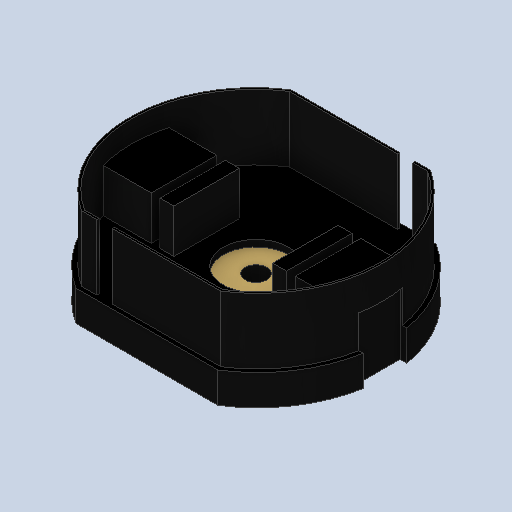
# Autodesk Inventor part: Base
Saved by Autodesk Inventor 2022.2 (Build 262287000, 287)
## iProperties
Created: 2021-01-16
Part Number: Base
Material: Ouro
Document SubType Name: Modeling
Designer: João
Density: 19.3 g/cm^3
Appearance: Suave - Preto
Mass: 3.82351 g
Surface Area: 5.41035 cm^2
Volume: 0.198109 cm^3
Author: João
Autodesk Inventor part; units mm, degrees
sketch "Esboço1" plane through (0, 0, 0) normal (0, 1, 0) x (-1, 0, 0)
  line L0 (3.25, 5) -> (-3.25, 5)
  line L1 (-3.25, -5) -> (3.25, -5)
  arc A0 (3.25, -5) -> (3.25, 5) centre (0.0795, 0) ccw
  arc A1 (-3.25, 5) -> (-3.25, -5) centre (-0.0795, 0) ccw
  line L2 (3.25, 5) -> (-3.25, 5)
  line L3 (-3.25, -5) -> (3.25, -5)
  line L4 (4.595, 3.8292) -> (-4.595, -3.8292) construction
  line L5 (-4.595, 3.8292) -> (4.595, -3.8292) construction
  line L6 (3.1014, -4.5) -> (-3.1014, -4.5)
  arc A2 (-3.1014, 4.5) -> (-3.1014, -4.5) centre (-0.0795, 0) ccw
  line L7 (-3.1014, 4.5) -> (3.1014, 4.5)
  arc A3 (3.1014, -4.5) -> (3.1014, 4.5) centre (0.0795, 0) ccw
  point P0 (0, 0)
  point P1 (0, 0)
  constraints: 16 end point, 12 point on circle, 4 centre point, 2 horizontal, 2 midpoint, 2 parallel
extrude "Extrusão1" add sketch "Esboço1" along normal blind 1.4 contours A0 L1 A1 L0 | L6 A2 L7 A3
sketch "Esboço13" plane through (0, 1.4, 0) normal (0, 1, 0) x (1, 0, 0)
  line L0 (-3.25, -5) -> (3.25, -5)
  arc A0 (3.25, -5) -> (3.25, 5) centre (0.0795, 0) ccw
  line L1 (3.25, 5) -> (-3.25, 5)
  arc A1 (-3.25, 5) -> (-3.25, -5) centre (-0.0795, 0) ccw
  line L2 (-3.1914, 4.8) -> (3.1914, 4.8)
  arc A2 (3.1914, -4.8) -> (3.1914, 4.8) centre (0.0795, 0) ccw
  line L3 (3.1914, -4.8) -> (-3.1914, -4.8)
  arc A3 (-3.1914, 4.8) -> (-3.1914, -4.8) centre (-0.0795, 0) ccw
  line L4 (3.25, 5) -> (-3.25, 5) projected
  line L5 (0.6483, 5) -> (-0.6517, 5)
  line L6 (-0.6517, 5) -> (-0.6517, 4.8)
  line L7 (-0.6517, 4.8) -> (0.6483, 4.8)
  line L8 (0.6483, 4.8) -> (0.6483, 5)
  line L9 (3.1617, 4.7) -> (-3.1617, 4.7)
  arc A4 (-3.1617, 4.7) -> (-3.1617, -4.7) centre (-0.0795, 0) ccw
  line L10 (-3.1617, -4.7) -> (3.1617, -4.7)
  arc A5 (3.1617, -4.7) -> (3.1617, 4.7) centre (0.0795, 0) ccw
  line L11 (-0.0017, 4.8) -> (-0.0017, 5)
  point P0 (0.6483, 4.8)
  dimension "d45" = 1.3
  constraints: 22 end point, 12 point on circle, 7 centre point, 2 midpoint, 2 parallel, 2 point on line, 1 horizontal, 1 perpendicular
  measures "d45" distance of L7.end L6.end
extrude "Extrusão13" add sketch "Esboço13" along normal blind 3 contours L2 A2 L3 A3
sketch "Esboço14" plane through (0, 4.4, 0) normal (0, 1, 0) x (1, 0, 0)
  line L0 (-3.1914, 4.8) -> (3.1914, 4.8) projected
  line L1 (3.1914, 4.8) -> (2.4914, 4.8)
  line L2 (3.1617, 4.7) -> (-3.1617, 4.7) projected
  line L3 (2.4914, 4.8) -> (1.7914, 4.8)
  line L4 (1.7914, 4.8) -> (1.7914, 4.7)
  line L5 (1.7914, 4.7) -> (2.4914, 4.7)
  line L6 (2.4914, 4.7) -> (2.4914, 4.8)
  arc A0 (-3.1914, 4.8) -> (-3.1914, -4.8) centre (-0.0795, 0) ccw projected
  line L7 (-3.1914, -4.8) -> (-2.4914, -4.8)
  line L8 (-3.1914, -4.8) -> (3.1914, -4.8) projected
  line L9 (3.1617, -4.7) -> (-3.1617, -4.7) projected
  line L10 (-2.4914, -4.8) -> (-1.7914, -4.8)
  line L11 (-1.7914, -4.8) -> (-1.7914, -4.7)
  line L12 (-1.7914, -4.7) -> (-2.4914, -4.7)
  line L13 (-2.4914, -4.7) -> (-2.4914, -4.8)
  point P0 (0, 0)
  point P1 (0.75, 4.8)
  dimension "d48" = 0.7
  dimension "d49" = 0.7
  dimension "d50" = 0.7
  dimension "d51" = 0.7
  constraints: 20 end point, 4 parallel, 4 point on line, 2 horizontal, 2 perpendicular
  measures "d48" distance of L0.end L1.end
  measures "d49" distance of L5.end L4.end
  measures "d50" distance of L7.start L7.end
  measures "d51" distance of L12.end L11.end
extrude "Extrusão14" cut sketch "Esboço14" against normal blind 3
extrude "Extrusão15" add sketch "Esboço13" along normal blind 1 contours L1 L11 L2 L6 | L8 L2 L11 L1
ref_plane "Plano de trabalho3" through (6, 0, 0) normal (1, 0, 0) x (0, 1, 0)
sketch "Esboço15" plane through (6, 0, 0) normal (1, 0, 0) x (0, 1, 0)
  line L0 (0, 1) -> (2.4, 1)
  line L1 (2.4, 1) -> (2.4, -1)
  line L2 (2.4, -1) -> (0, -1)
  line L3 (0, -1) -> (0, 1)
  point P0 (0, 0)
  dimension "d56" = 2
  constraints: 8 end point, 2 parallel, 1 horizontal, 1 perpendicular
  measures "d56" distance of L0.end L1.end
ref_plane "Plano de trabalho4" through (-6, 0, 0) normal (-1, 0, 0) x (0, -1, 0)
sketch "Esboço16" plane through (-6, 0, 0) normal (-1, 0, 0) x (0, -1, 0)
  line L0 (-2.4, -1) -> (0, -1)
  line L1 (-2.4, 1) -> (-2.4, -1)
  line L2 (0, 1) -> (-2.4, 1)
  line L3 (0, -1) -> (0, 1)
  point P0 (0, 0)
  constraints: 8 end point
ref_plane "Plano de trabalho5" through (-5.7, 4.4, 0) normal (1, 0, 0) x (0, 1, 0)
sketch "Esboço17" plane through (-5.7, 4.4, 0) normal (1, 0, 0) x (0, 1, 0)
  line L0 (-3, -4.7) -> (-3, 4.7) projected
  line L1 (-3, 1.5) -> (-1, 1.5)
  line L2 (-1, 1.5) -> (-1, -1.5)
  line L3 (-1, -1.5) -> (-3, -1.5)
  line L4 (-3, -1.5) -> (-3, 1.5)
  point P0 (-4.4, 0)
  dimension "d57" = 2
  dimension "d58" = 3
  constraints: 8 end point, 2 parallel, 1 horizontal, 1 perpendicular, 1 point on line
  measures "d57" distance of L2.end L3.end
  measures "d58" distance of L1.end L2.end
extrude "Extrusão16" add sketch "Esboço17" along normal blind 3.537
ref_plane "Plano de trabalho6" through (5.7, 4.4, 0) normal (-1, 0, 0) x (0, -1, 0)
sketch "Esboço18" plane through (5.7, 4.4, 0) normal (-1, 0, 0) x (0, -1, 0)
  line L0 (1, 1.5) -> (3, 1.5) projected
  line L1 (3, -1.5) -> (3, 1.5) projected
  line L2 (3, -1.5) -> (1, -1.5) projected
  line L3 (1, -1.5) -> (1, 1.5) projected
  point P0 (4.4, 0)
extrude "Extrusão17" add sketch "Esboço18" along normal blind 3.537
sketch "Esboço20" plane through (2.163, 3.4, -1.5) normal (0, 1, 0) x (1, 0, 0)
  circle A0 centre (-2.163, -1.5) radius 1.5
  line L0 (-7.6591, 0) -> (-4.326, 0) projected
  line L1 (-4.326, -3) -> (-7.6591, -3) projected
  line L2 (-5.063, 0) -> (-5.463, 0)
  line L3 (-5.463, 0) -> (-5.463, -3)
  line L4 (-5.463, -3) -> (-5.063, -3)
  line L5 (-5.063, -3) -> (-5.063, 0)
  line L6 (-5.263, 0) -> (-5.263, -3)
  line L7 (-7.6591, 0) -> (-4.326, 0) projected
  line L8 (-7.6591, -3) -> (-4.326, -3) projected
  line L9 (-4.326, 0) -> (-4.426, 0)
  line L10 (-4.426, 0) -> (-4.426, -3)
  line L11 (-4.426, -3) -> (-4.326, -3)
  line L12 (-4.326, -3) -> (-4.326, 0)
  line L13 (-2.163, -4.6901) -> (-2.163, 0.7868)
  line L14 (3.3331, 0) -> (0, 0)
  line L15 (0, -3) -> (3.3331, -3)
  line L16 (0.737, 0) -> (1.137, 0)
  line L17 (1.137, 0) -> (1.137, -3)
  line L18 (1.137, -3) -> (0.737, -3)
  line L19 (0.737, -3) -> (0.737, 0)
  line L20 (0.937, 0) -> (0.937, -3)
  line L21 (3.3331, 0) -> (0, 0)
  line L22 (3.3331, -3) -> (0, -3)
  line L23 (0, 0) -> (0.1, 0)
  line L24 (0.1, 0) -> (0.1, -3)
  line L25 (0.1, -3) -> (0, -3)
  line L26 (0, -3) -> (0, 0)
  line L27 (0.737, -2.5) -> (1.137, -2.5)
  line L28 (1.137, -2.5) -> (1.137, -0.5)
  line L29 (1.137, -0.5) -> (0.737, -0.5)
  line L30 (0.737, -0.5) -> (0.737, -2.5)
  line L31 (0.737, -2.5) -> (1.137, -0.5) construction
  line L32 (1.137, -2.5) -> (0.737, -0.5) construction
  line L33 (-5.463, -2.5) -> (-5.063, -2.5)
  line L34 (-5.063, -2.5) -> (-5.063, -0.5)
  line L35 (-5.063, -0.5) -> (-5.463, -0.5)
  line L36 (-5.463, -0.5) -> (-5.463, -2.5)
  line L37 (-5.463, -2.5) -> (-5.063, -0.5) construction
  line L38 (-5.063, -2.5) -> (-5.463, -0.5) construction
  point P0 (-2.163, -1.5)
  point P1 (-5.463, 0)
  point P2 (1.137, 0)
  point P3 (0.937, -1.5)
  point P4 (-5.263, -1.5)
  point P5 (0.737, -0.5)
  point P6 (0.737, -2.5)
  point P7 (1.137, -2.5)
  dimension "d68" = 3
  dimension "d69" = 0.4
  dimension "d70" = 3.1
  dimension "d71" = 0.1
  dimension "d101" = 2
  constraints: 70 end point, 13 symmetric about line, 9 point on line, 8 midpoint, 8 parallel, 4 horizontal, 4 perpendicular, 1 centre point, 1 coincident, 1 vertical
  measures "d68" diameter of A0
  measures "d69" distance of L4.end L3.end
  measures "d70" distance from line of L6 point (-2.163, -1.5)
  measures "d71" distance of L11.end L10.end
  measures "d101" distance of L28.end L27.end
extrude "Extrusão18" cut sketch "Esboço20" against normal blind 2 contours L0 L12 L1 L10 | L24 L15 L26 L14
extrude "Extrusão19" cut sketch "Esboço20" against normal blind 3.4 contours L35 L6 L33 L3 | L35 L5 L33 L6 | L17 L27 L20 L29 | L20 L27 L19 L29
sketch "Esboço21" plane through (0, 1.4, 0) normal (0, 1, 0) x (1, 0, 0)
  circle A0 centre (0, 0) radius 1.5
  circle A1 centre (0, 0) radius 0.5
  dimension "d76" = 3
  dimension "d79" = 1
  constraints: 2 centre point, 2 coincident
  measures "d76" diameter of A0
  measures "d79" diameter of A1
extrude "Extrusão20" cut sketch "Esboço21" against normal blind 0.3 contours A0 | A1
extrude "Extrusão21" cut sketch "Esboço21" against normal blind 1.55 contours A1
sketch "Esboço22" plane through (-5.7, 3.4, 1.5) normal (0, 1, 0) x (1, 0, 0)
  arc A0 (0.1002, 3) -> (0, 2.5649) centre (5.6205, 1.5) ccw projected
  line L0 (0, 3) -> (0.1002, 3) projected
  line L1 (0, 3) -> (0, 2.5649) projected
  arc A1 (0, 0.4351) -> (0.1002, 0) centre (5.6205, 1.5) ccw projected
  line L2 (0, 0.4351) -> (0, 0) projected
  line L3 (0, 0) -> (0.1002, 0) projected
  arc A2 (11.4, 2.5649) -> (11.2998, 3) centre (5.7795, 1.5) ccw projected
  line L4 (11.4, 2.5649) -> (11.4, 3) projected
  line L5 (11.4, 3) -> (11.2998, 3) projected
  arc A3 (11.2998, 0) -> (11.4, 0.4351) centre (5.7795, 1.5) ccw projected
  line L6 (11.4, 0) -> (11.2998, 0) projected
  line L7 (11.4, 0) -> (11.4, 0.4351) projected
  point P0 (5.7, 1.5)
extrude "Extrusão22" cut sketch "Esboço22" against normal blind 2
sketch "Esboço23" plane through (0, 0, 0) normal (0, -1, 0) x (1, 0, 0)
  circle A0 centre (0, 0) radius 0.5 projected
  circle A1 centre (0, 0) radius 2.5
  dimension "d84" = 5
  constraints: 1 centre point, 1 coincident
  measures "d84" diameter of A1
extrude "Extrusão23" add sketch "Esboço23" along normal blind 0.8
ref_plane "Plano de trabalho7" through (-6, 1.4, 0) normal (-1, 0, 0) x (0, -1, 0)
ref_plane "Plano de trabalho8" through (6, 1.4, 0) normal (1, 0, 0) x (0, 1, 0)
sketch "Esboço24" plane through (-6, 1.4, 0) normal (-1, 0, 0) x (0, -1, 0)
  line L0 (1.4, 0) -> (-1.5, 0)
  line L1 (1.4, 5) -> (1.4, -5) projected
  line L2 (1.4, -1) -> (-1.5, -1)
  line L3 (-1.5, -1) -> (-1.5, 1)
  line L4 (-1.5, 1) -> (1.4, 1)
  line L5 (1.4, 1) -> (1.4, -1)
  dimension "d87" = 2.9
  dimension "d88" = 2
  dimension "d89" = 2.9
  constraints: 10 end point, 2 horizontal, 2 parallel, 1 perpendicular, 1 point on line
  measures "d87" distance of L0.start L0.end
  measures "d88" distance of L2.end L3.end
  measures "d89" distance between parallel lines of L1 L3
extrude "Extrusão24" cut sketch "Esboço24" against normal blind 0.4
sketch "Esboço25" plane through (6, 1.4, 0) normal (1, 0, 0) x (0, 1, 0)
  line L0 (1.5, -1) -> (1.5, 1) projected
  line L1 (-1.4, -1) -> (1.5, -1) projected
  line L2 (-1.4, 1) -> (-1.4, -1) projected
  line L3 (1.5, 1) -> (-1.4, 1) projected
  point P0 (-1.4, 0)
extrude "Extrusão25" cut sketch "Esboço25" against normal blind 0.4
extrude "Extrusão26" cut sketch "Esboço20" against normal blind 2 contours L0 L6 L35 L3 | L0 L5 L35 L6 | L33 L6 L1 L3 | L33 L5 L1 L6 | L17 L29 L20 L14 | L20 L29 L19 L14 | L17 L15 L20 L27 | L20 L15 L19 L27
